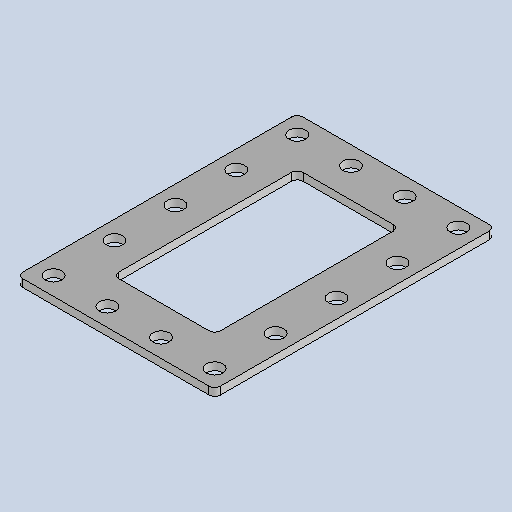
# Autodesk Inventor part: PRS 9606 charging flange round_D1200 940
Saved by Autodesk Inventor 2026.2 (Build 302298010, 298A)
## iProperties
Created: 2025-02-13
Part Number: PRS 9606 charging flange round_D1200 940
Material: Steel
Document SubType Name: Sheet Metal
Designer: admin
Mass: 2237.08 g
Surface Area: 894.773 cm^2
Volume: 284.978 cm^3
Density: 7.85 g/cm^3
Flat Pattern Width: 29.2 cm
Flat Pattern Length: 20.6 cm
Flat Pattern Area: 601.52 cm^2
Sheet Metal Rule: AISI304 4mm Die 32
Sheet Metal Width: 292,000 mm
Sheet Metal Length: 206,000 mm
Sheet Metal Area: 60152,000 mm^2
Appearance: Default
Author: pokla
Autodesk Inventor part; units mm, degrees
ref_plane "YZ Plane" through (0, 0, 0) normal (1, 0, 0) x (0, 1, 0)
ref_plane "XZ Plane" through (0, 0, 0) normal (0, 1, 0) x (-1, 0, 0)
ref_plane "XY Plane" through (0, 0, 0) normal (0, 0, 1) x (1, 0, 0)
sketch "Sketch2" plane through (0, 0, 0) normal (0, 0, 1) x (1, 0, 0)
  line L0 (-53, -96) -> (53, -96)
  line L1 (53, -96) -> (53, 96)
  line L2 (53, 96) -> (-53, 96)
  line L3 (-53, 96) -> (-53, -96)
  line L4 (-53, -96) -> (53, 96) construction
  line L5 (53, -96) -> (-53, 96) construction
  line L6 (-103, -146) -> (103, -146)
  line L7 (103, -146) -> (103, 146)
  line L8 (103, 146) -> (-103, 146)
  line L9 (-103, 146) -> (-103, -146)
  point P0 (0, 0)
  dimension "d29" = 106
  dimension "d30" = 192
  dimension "d31" = 50
  measures "d29" distance of L2.end L1.end
  measures "d30" distance of L1.end L0.end
  measures "d31" distance between parallel lines of L3 L9
extrude "Plate2" add sketch "Sketch2" along normal blind 8
sketch "Sketch5" plane through (0, 0, 8) normal (0, 0, 1) x (1, 0, 0)
  line L0 (53, 96) -> (53, -96) construction
  line L1 (53, -96) -> (-53, -96) construction
  line L2 (-53, -96) -> (-53, 96) construction
  line L3 (-53, 96) -> (53, 96) construction
  line L4 (103, -146) -> (-103, -146) construction
  line L5 (103, 146) -> (103, -146) construction
  line L6 (-103, 146) -> (103, 146) construction
  line L7 (-103, -146) -> (-103, 146) construction
  line L8 (-84, 127) -> (84, 127) construction
  line L9 (84, 127) -> (84, -127) construction
  line L10 (84, -127) -> (-84, -127) construction
  line L11 (-84, -127) -> (-84, 127) construction
  line L12 (-53, 0) -> (53, 0) construction
  line L13 (0, 96) -> (0, -96)
  point P0 (0, 0)
  point P1 (0, -127)
  point P2 (-84, 63.5)
  point P3 (-84, 0)
  point P4 (-84, -63.5)
  point P5 (-28, -127)
  point P6 (28, -127)
  point P7 (84, -63.5)
  point P8 (84, 0)
  point P9 (84, 63.5)
  point P10 (28, 127)
  point P11 (-28, 127)
  dimension "d34" = 19
  dimension "d49" = 63.5
  dimension "d50" = 63.5
  dimension "d51" = 56
  dimension "d52" = 56
  dimension "d53" = 56
  constraints: 12 end point, 8 point on line, 7 midpoint, 4 coincident, 3 symmetric about line, 2 vertical alignment, 1 horizontal alignment, 3 other
  measures "d34" distance between parallel lines of L4 L10
  measures "d49" distance of point (-84, 63.5) point (-84, 127)
  measures "d50" distance of point (-84, 0) point (-84, 63.5)
  measures "d51" distance of point (-28, 127) point (-84, 127)
  measures "d52" distance of point (28, 127) point (-28, 127)
  measures "d53" distance of point (84, 127) point (28, 127)
fillet "Corner Round1" radius 6 8 edges at (-103, -146, 4) (-103, 146, 4) (103, 146, 4) (103, -146, 4) (53, -96, 4) (-53, -96, 4) (-53, 96, 4) (53, 96, 4)
hole "Hole1" at (-84, 127, 8) at (-84, 63.5, 8) at (-84, 0, 8) at (-84, -63.5, 8) at (-84, -127, 8) at (-28, -127, 8) at (28, -127, 8) at (84, -127, 8) at (84, -63.5, 8) at (84, 0, 8) at (84, 63.5, 8) at (84, 127, 8) at (28, 127, 8) at (-28, 127, 8) direction (0, 0, -1) diameter 17 end through all
equation "\"d49\" = d50"
equation "\"d51\" = d53"
equation "\"d52\" = d53"
equation "\"d29\" = ChargingHatch_hight - 2 * Thickness"
equation "\"d30\" = ChargingHatch_width - 2 * Thickness"
equation "\"d59\" = Thickness"
equation "\"d14\" = Thickness"
equation "\"BendReliefWidth\" = Thickness"
equation "\"BendReliefDepth\" = 0.5 * Thickness"
equation "\"CornerReliefSize\" = 4 * Thickness"
equation "\"MinimumRemnant\" = 2 * Thickness"
equation "\"TransitionRadius\" = BendRadius"
equation "\"JacobiRadiusSize\" = BendRadius"
equation "\"GapSize\" = Thickness"
equation "\"ChargingHatch_hight\" = 122"
equation "\"Thickness\" = 8"
equation "\"ChargingHatch_width\" = 208"
equation "\"BendRadius\" = 6"
body "Solid3"
